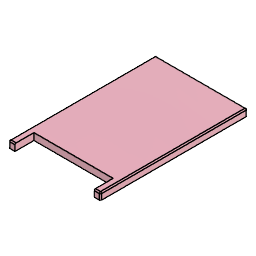
top_plate (Autodesk Fusion 360 design; units mm, degrees)
part number: 2025-10-01-09-24-30-311
Autodesk Fusion 360 part; units mm, degrees
sketch "Top Plate" plane through (0, 0, 0) normal (0, 0, 1) x (1, 0, 0)
  line L0 (0, 0) -> (160, 0)
  line L1 (160, 0) -> (160, 256)
  line L2 (160, 256) -> (0, 256)
  line L3 (0, 256) -> (0, 0)
  line L4 (11, 0) -> (149, 0)
  line L5 (149, 0) -> (149, 33)
  line L6 (149, 33) -> (11, 33)
  line L7 (11, 33) -> (11, 0)
  dimension "d4" = 160
  dimension "d5" = 256
  dimension "d12" = 33
  dimension "d14" = 11
  dimension "d15" = 11
  constraint horizontal L0
  constraint vertical L1
  constraint horizontal L2
  constraint vertical L3
  constraint coincident L0.start L3.end
  constraint horizontal L4
  constraint vertical L5
  constraint horizontal L6
  constraint vertical L7
  constraint coincident L0 L4.start
  measures "d4" distance of L0.start L0.end
  measures "d5" distance of L0.end L1.end
  measures "d12" distance of L0 L6
  measures "d14" distance of L1 L5
  measures "d15" distance of L3 L7
extrude "Extrude1" add sketch "Top Plate" along normal blind 12 contours L0 L1 L2 L3 L5 L6 L7
fillet "Fillet2" radius 2 9 edges at (0, 0, 6) (160, 0, 6) (160, 256, 6) (0, 256, 6) (0, 128, 12) (80, 256, 12) (160, 128, 12) (5.5, 0, 12) (154.5, 0, 12)
equation "block_size = 16 mm" comment "The size of the blocks used for the dimensions of the Minecraft Pig."
equation "fillet_radius = 2 mm" comment "The radius of the fillets applied to the Top Plate."
equation "pine_thickness = 12 mm" comment "The thickness of the pine boards used for the Minecraft Pig's body."
equation "d4 = 10 * block_size"
equation "d5 = 16 * block_size"
equation "d6 = pine_thickness"
equation "tolerance = 1 mm" comment "The tolerance to add to the cutaway for the Minecraft Pig's face."
equation "cutaway_length = 2 * block_size + tolerance" comment "The length of the cutaway for the Minecraft Pig's face."
equation "d12 = cutaway_length"
equation "cutaway_side_width = pine_thickness - tolerance" comment "The width of the wood at the size of the cutaway for the Minecraft Pig's face."
equation "d14 = cutaway_side_width"
equation "d15 = cutaway_side_width"
equation "d17 = fillet_radius"
named bodies: "Top Plate"
